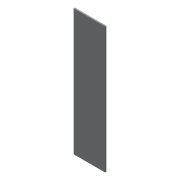
# Autodesk Inventor part: grippy
Saved by Autodesk Inventor 2018 (Build 220112000, 112)
## iProperties
Created: 2017-12-20
Part Number: grippy
Material: Generic
Document SubType Name: Modeling
Designer: dsayers
Density: 1 g/cm^3
Appearance: Default
Author: dsayers
Autodesk Inventor part; units mm, degrees
ref_plane "YZ Plane" through (0, 0, 0) normal (1, 0, 0) x (0, 1, 0)
ref_plane "XZ Plane" through (0, 0, 0) normal (0, 1, 0) x (-1, 0, 0)
ref_plane "XY Plane" through (0, 0, 0) normal (0, 0, 1) x (1, 0, 0)
sketch "Sketch1" plane through (0, 0, 0) normal (0, 0, 1) x (1, 0, 0)
  line L0 (0, 0) -> (57.15, 0)
  line L1 (57.15, 0) -> (57.15, 304.8)
  line L2 (57.15, 304.8) -> (0, 304.8)
  line L3 (0, 304.8) -> (0, 0)
  dimension "d0" = 304.8
  dimension "d1" = 57.15
  constraints: 8 end point, 2 parallel, 1 horizontal, 1 perpendicular
  measures "d0" distance of L0.end L1.end
  measures "d1" distance of L1.end L2.end
extrude "Extrusion1" add sketch "Sketch1" along normal blind 3.175
sketch "Sketch2" plane through (0, 0, 0) normal (0, 0, -1) x (-1, 0, 0)
  circle A0 centre (-9.525, 245.6024) radius 2.2479 projected
  circle A1 centre (-28.575, 245.6024) radius 2.2479 projected
  circle A2 centre (-47.625, 245.6024) radius 2.2479 projected
  circle A3 centre (-9.525, 99.2024) radius 2.2479 projected
  circle A4 centre (-28.575, 99.2024) radius 2.2479 projected
  circle A5 centre (-47.625, 99.2024) radius 2.2479 projected
  point P0 (0, 0)
sketch "Sketch3" plane through (0, 0, 0) normal (0, 0, -1) x (-1, 0, 0)
  point P0 (0, 0)
  point P1 (-47.625, 99.2024)
  point P2 (-28.575, 99.2024)
  point P3 (-9.525, 99.2024)
  point P4 (-47.625, 245.6024)
  point P5 (-28.575, 245.6024)
  point P6 (-9.525, 245.6024)
hole "Hole1" at (47.625, 99.2024, 0) at (28.575, 99.2024, 0) at (9.525, 99.2024, 0) at (47.625, 245.6024, 0) at (28.575, 245.6024, 0) at (9.525, 245.6024, 0) direction (0, 0, 1) diameter 4.4958 depth 25.4 tip angle 118 clearance for "Flat Head Machine Screw (82)" size "#8" standard "Ansi Unified Screw Threads"
sketch "Sketch4" plane through (0, 0, 3.175) normal (0, 0, 1) x (1, 0, 0)
  circle A0 centre (47.625, 99.2024) radius 2.2479 projected
  circle A1 centre (28.575, 99.2024) radius 2.2479 projected
  circle A2 centre (9.525, 99.2024) radius 2.2479 projected
  line L0 (0, 0) -> (57.15, 0) projected
  line L1 (0, 304.8) -> (0, 0) projected
  point P0 (19.05, 12.7)
  point P1 (38.1, 12.7)
  point P2 (19.05, 38.1)
  point P3 (38.1, 38.1)
  point P4 (19.05, 63.5)
  point P5 (38.1, 63.5)
  point P6 (19.05, 88.9)
  point P7 (38.1, 88.9)
  point P8 (19.05, 114.3)
  point P9 (38.1, 114.3)
  point P10 (19.05, 139.7)
  point P11 (38.1, 139.7)
  point P12 (19.05, 165.1)
  point P13 (38.1, 165.1)
  point P14 (19.05, 190.5)
  point P15 (38.1, 190.5)
  point P16 (19.05, 215.9)
  point P17 (38.1, 215.9)
  point P18 (19.05, 241.3)
  point P19 (38.1, 241.3)
  point P20 (19.05, 266.7)
  point P21 (38.1, 266.7)
  point P22 (19.05, 292.1)
  point P23 (38.1, 292.1)
  dimension "d11" = 9.525
  dimension "d12" = 9.525
  dimension "d13" = 9.525
  dimension "d14" = 9.525
  dimension "d15" = 12.7
  dimension "d16" = 12.7
  dimension "d19" = 25.4
  constraints: 1 vertical, 22 other
  measures "d11" horizontal distance of A0.centre point (38.1, 12.7)
  measures "d12" horizontal distance of A1.centre point (38.1, 12.7)
  measures "d13" horizontal distance of A1.centre point (19.05, 12.7)
  measures "d14" horizontal distance of A2.centre point (19.05, 12.7)
  measures "d15" distance from line of L0 point (38.1, 12.7)
  measures "d16" distance from line of L0 point (19.05, 12.7)
  measures "d19" distance of point (19.05, 12.7) point (19.05, 38.1)
hole "Hole2" at (19.05, 12.7, 3.175) at (38.1, 12.7, 3.175) at (19.05, 38.1, 3.175) at (38.1, 38.1, 3.175) at (19.05, 63.5, 3.175) at (38.1, 63.5, 3.175) at (19.05, 88.9, 3.175) at (38.1, 88.9, 3.175) at (19.05, 114.3, 3.175) at (38.1, 114.3, 3.175) at (19.05, 139.7, 3.175) at (38.1, 139.7, 3.175) at (19.05, 165.1, 3.175) at (38.1, 165.1, 3.175) at (19.05, 190.5, 3.175) at (38.1, 190.5, 3.175) at (19.05, 215.9, 3.175) at (38.1, 215.9, 3.175) at (19.05, 241.3, 3.175) at (38.1, 241.3, 3.175) at (19.05, 266.7, 3.175) at (38.1, 266.7, 3.175) at (19.05, 292.1, 3.175) at (38.1, 292.1, 3.175) direction (0, 0, -1) diameter 4.4958 depth 25.4 tip angle 118 clearance for "Flat Head Machine Screw (82)" size "#8" standard "Ansi Unified Screw Threads"
equation "\"d11\" = d12"
equation "\"d13\" = d14"
equation "\"d16\" = d15"
body "Solid1"
